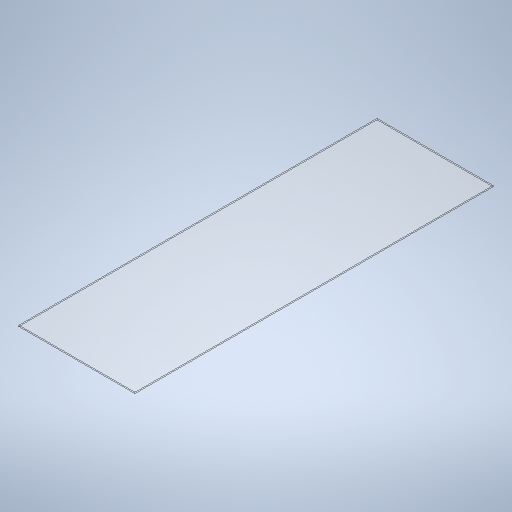
# Autodesk Inventor part: roof
Saved by Autodesk Inventor 2025 (Build 290162010, 162A)
## iProperties
Created: 2024-06-14
Part Number: roof
Material: Aluminum 6061
Document SubType Name: Modeling
Designer: Alan Thomas
Mass: 9590.4 g
Surface Area: 14404 cm^2
Volume: 3552 cm^3
Density: 2.7 g/cm^3
Appearance: Polycarbonate - Clear
Author: Alan Thomas
Autodesk Inventor part; units mm, degrees
ref_plane "YZ Plane" through (0, 0, 0) normal (1, 0, 0) x (0, 1, 0)
ref_plane "XZ Plane" through (0, 0, 0) normal (0, 1, 0) x (-1, 0, 0)
ref_plane "XY Plane" through (0, 0, 0) normal (0, 0, 1) x (1, 0, 0)
sketch "Sketch1" plane through (0, 0, 0) normal (0, 1, 0) x (-1, 0, 0)
  line L0 (0, 0) -> (480, 0)
  line L1 (480, 0) -> (480, -1480)
  line L2 (480, -1480) -> (0, -1480)
  line L3 (0, -1480) -> (0, 0)
  dimension "d0" = 480
  dimension "d1" = 1480
  constraints: 8 end point, 2 parallel, 1 horizontal, 1 perpendicular
  measures "d0" distance of L1.end L2.end
  measures "d1" distance of L0.end L1.end
extrude "Extrusion1" add sketch "Sketch1" along normal blind 5
body "Solid1"
